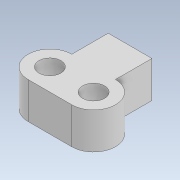
# Autodesk Inventor part: 夹爪连接件
Saved by Autodesk Inventor 2022.5 (Build 265521000, 521)
## iProperties
Created: 2024-11-12
Part Number: 夹爪连接件
Material: 常规
Document SubType Name: Modeling
Designer: Gagouking
Density: 1 g/cm^3
Appearance: 默认
Author: Gagouking
Autodesk Inventor part; units mm, degrees
ref_plane "YZ Plane" through (0, 0, 0) normal (1, 0, 0) x (0, 1, 0)
ref_plane "XZ Plane" through (0, 0, 0) normal (0, 1, 0) x (-1, 0, 0)
ref_plane "XY Plane" through (0, 0, 0) normal (0, 0, 1) x (1, 0, 0)
sketch "草图1" plane through (0, 0, 0) normal (0, 1, 0) x (-1, 0, 0)
  line L0 (0, 0) -> (-6, 0) construction
  line L1 (0, 3) -> (-6, 3)
  line L2 (-6, -3) -> (0, -3)
  arc A0 (0, -3) -> (0, 3) centre (0, 0) ccw
  arc A1 (-6, 3) -> (-6, -3) centre (-6, 0) ccw
  circle A2 centre (0, 0) radius 1.5
  circle A3 centre (-6, 0) radius 1.5
  point P0 (-3, 0)
  dimension "d0" = 6
  dimension "d1" = 3
  dimension "d2" = 3
  dimension "d3" = 1.5
  constraints: 8 end point, 4 centre point, 4 point on circle, 4 tangent, 2 coincident, 1 horizontal, 1 midpoint, 1 parallel
  measures "d0" distance of L0.start L0.end
  measures "d1" diameter of A2
  measures "d2" diameter of A3
  measures "d3" radial gap between concentric circles of A2 A0
extrude "拉伸1" add sketch "草图1" along normal blind 5
sketch "草图2" plane through (6, 0, -3) normal (0, 0, -1) x (-1, 0, 0)
  line L0 (0, 0) -> (6, 0) projected
  line L1 (6, 0) -> (6, 5) projected
  line L2 (0, 5) -> (6, 5) projected
  line L3 (0, 0) -> (0, 5) projected
  line L4 (0, 0) -> (6, 0)
  line L5 (6, 0) -> (6, 5)
  line L6 (6, 5) -> (0, 5)
  line L7 (0, 5) -> (0, 0)
  line L8 (0, 0) -> (6, 5) construction
  line L9 (6, 0) -> (0, 5) construction
  line L10 (0, 5) -> (6, 5) projected
  line L11 (6, 0) -> (6, 5) projected
  line L12 (0, 0) -> (6, 0) projected
  line L13 (0, 0) -> (0, 5) projected
  circle A0 centre (3, 2.5) radius 1.5
  dimension "d6" = 3
  constraints: 12 end point, 4 collinear, 2 midpoint, 2 parallel, 1 centre point, 1 coincident, 1 horizontal, 1 perpendicular
  measures "d6" diameter of A0
extrude "拉伸2" add sketch "草图2" along normal blind 5
